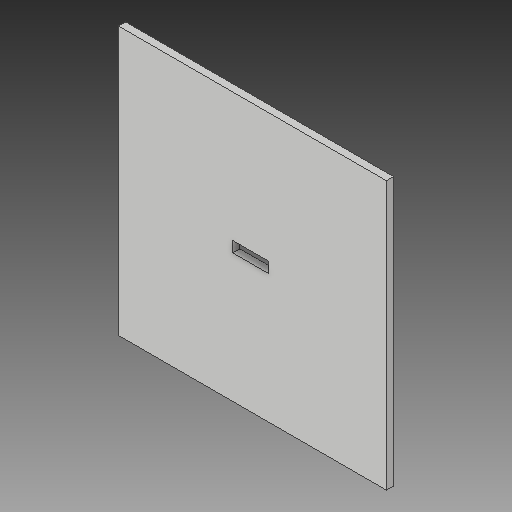
# Autodesk Inventor part: Pièce-moteur-vis_CPY1
Saved by Autodesk Inventor 2019 (Build 230136000, 136)
## iProperties
Created: 2018-12-30
Part Number: Pièce-moteur-vis_CPY1
Material: Générique
Document SubType Name: Modeling
Designer: pouey
Density: 1 g/cm^3
Appearance: Par défaut
Author: pouey
Autodesk Inventor part; units mm, degrees
ref_plane "YZ Plane" through (0, 0, 0) normal (1, 0, 0) x (0, 1, 0)
ref_plane "XZ Plane" through (0, 0, 0) normal (0, 1, 0) x (-1, 0, 0)
ref_plane "XY Plane" through (0, 0, 0) normal (0, 0, 1) x (1, 0, 0)
sketch "Esquisse1" plane through (0, 0, 0) normal (0, 0, 1) x (1, 0, 0)
  line L0 (0, 0) -> (75, 0)
  line L1 (75, 0) -> (75, 75)
  line L2 (75, 75) -> (0, 75)
  line L3 (0, 75) -> (0, 0)
  dimension "d0" = 75
  dimension "d1" = 75
  constraints: 8 end point, 2 parallel, 1 horizontal, 1 perpendicular
  measures "d0" distance of L1.end L2.end
  measures "d1" distance of L0.end L1.end
extrude "Extrusion1" add sketch "Esquisse1" along normal blind 2
sketch "Esquisse2" plane through (0, 0, 2) normal (0, 0, 1) x (1, 0, 0)
  line L0 (32, 36) -> (42, 36)
  line L1 (42, 36) -> (42, 39)
  line L2 (42, 39) -> (32, 39)
  line L3 (32, 39) -> (32, 36)
  line L4 (0, 0) -> (75, 0) projected
  line L5 (0, 75) -> (0, 0) projected
  dimension "d4" = 10
  dimension "d5" = 3
  dimension "d6" = 36
  dimension "d7" = 32
  constraints: 8 end point, 2 parallel, 1 horizontal, 1 perpendicular
  measures "d4" distance of L1.end L2.end
  measures "d5" distance of L0.end L1.end
  measures "d6" distance between parallel lines of L4 L0
  measures "d7" distance between parallel lines of L5 L3
extrude "Extrusion2" cut sketch "Esquisse2" against normal blind 2
